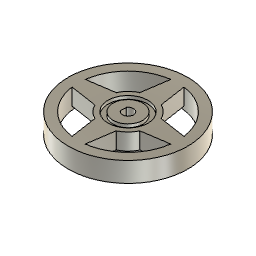
proto_wheel (Autodesk Fusion 360 design; units mm, degrees)
Autodesk Fusion 360 part; units mm, degrees
sketch "스케치1" plane through (0, 0, 0) normal (0, 0, 1) x (1, 0, 0)
  circle A0 centre (0, 0) radius 36
  dimension "d1" = 72
  constraint coincident A0.centre origin
  measures "d1" diameter of A0
extrude "돌출1" add sketch "스케치1" along normal blind 12 makes body 1
sketch "스케치2" plane through (0, 0, 12) normal (0, 0, 1) x (-1, 0, 0)
  circle A0 centre (0, 0) radius 36
  circle A1 centre (0, 0) radius 9
  circle A2 centre (0, 0) radius 12
  dimension "d4" = 18
  dimension "d5" = 24
  constraint concentric A0 A1
  constraint concentric A1 A2
  measures "d4" diameter of A1
  measures "d5" diameter of A2
extrude "돌출2" cut sketch "스케치2" against normal blind 2 contours A2 bodies 1
sketch "스케치3" plane through (0, 0, 12) normal (0, 0, 1) x (-1, 0, 0)
  circle A0 centre (0, 0) radius 9
  circle A1 centre (0, 0) radius 30
  line L0 (32, 0) -> (32, 4)
  line L1 (32, 0) -> (32, -4)
  line L2 (-4, -32) -> (0, -32)
  line L3 (4, -32) -> (0, -32)
  line L4 (-7, 9.744) -> (-4, 29.7321)
  circle A2 centre (0, 0) radius 12
  line L5 (-4, -29.7321) -> (-7, -9.7468)
  line L6 (4, -29.7321) -> (7, -9.7468)
  line L7 (29.7321, -4) -> (9.7468, -7)
  line L8 (29.7321, 4) -> (9.7468, 7)
  line L9 (-9.7468, -7) -> (-29.7321, -4)
  line L10 (4, 32) -> (0, 32)
  line L11 (7, 9.7468) -> (4, 29.7321)
  line L12 (0, 4) -> (0, 0)
  line L13 (0, 7) -> (0, 0)
  line L14 (-9.7468, 7) -> (-29.7321, 4)
  circle A3 centre (0, 0) radius 15
  dimension "d43" = 4
  dimension "d45" = 7
  dimension "d46" = 30
  constraint concentric A0 A1
  constraint vertical L0
  constraint vertical L1
  constraint horizontal L2
  constraint horizontal L3
  constraint coincident A1 L4.end
  constraint coincident A1 L5.start
  constraint coincident A2 L5.end
  constraint coincident A1 L6.start
  constraint coincident A2 L6.end
  constraint coincident A1 L7.start
  constraint coincident A2 L7.end
  constraint coincident A1 L8.start
  constraint coincident A2 L8.end
  constraint coincident A2 L9.start
  constraint coincident A1 L9.end
  constraint horizontal L10
  constraint coincident A2 L11.start
  constraint coincident A1 L11.end
  constraint vertical L12
  constraint coincident A0.centre A1.centre
  constraint vertical L13
  constraint coincident A2 L14.start
  constraint coincident A1 L14.end
  constraint concentric A2 A3
  measures "d43" distance of A0.centre L12.start
  measures "d45" distance of A0.centre L13.start
  measures "d46" diameter of A3
extrude "돌출3" cut sketch "스케치3" against normal blind 12 contours A1 L8 L11 A3 | A1 L6 L7 A3 | A1 L4 L14 A3 | A1 L5 L9 A3 bodies 1
sketch "스케치4" plane through (0, 0, 12) normal (0, 0, 1) x (-1, 0, 0)
  circle A0 centre (0, 0) radius 9
  circle A1 centre (0, 0) radius 3.5
  dimension "d49" = 7
  constraint coincident A0.centre A1.centre
  measures "d49" diameter of A1
extrude "돌출4" cut sketch "스케치4" against normal blind 12 contours A1 bodies 1
sketch "스케치5" plane through (0, 0, 12) normal (0, 0, 1) x (-1, 0, 0)
  circle A0 centre (0, 0) radius 3.5
  circle A1 centre (0, 0) radius 9
  circle A2 centre (0, 0) radius 30
  circle A3 centre (0, 0) radius 3.5
  dimension "d52" = 60
  constraint coincident A0.centre A1.centre
  measures "d52" diameter of A2
sketch "스케치6" plane through (0, 0, 0) normal (0, 0, -1) x (1, 0, 0)
  circle A0 centre (0, 0) radius 3.5
  line L0 (-4, 29.7321) -> (-6.4287, 13.5525)
  arc A1 (-6.4287, 13.5525) -> (-13.5525, 6.4287) centre (0, 0) ccw
  line L1 (-13.5525, 6.4287) -> (-29.7321, 4)
  arc A2 (-4, 29.7321) -> (-29.7321, 4) centre (0, 0) ccw
  arc A3 (29.7321, 4) -> (4, 29.7321) centre (0, 0) ccw
  line L2 (29.7321, 4) -> (13.5525, 6.4287)
  arc A4 (13.5525, 6.4287) -> (6.4284, 13.5527) centre (0, 0) ccw
  line L3 (6.4284, 13.5527) -> (4, 29.7321)
  arc A5 (-13.5525, -6.4287) -> (-6.4287, -13.5525) centre (0, 0) ccw
  line L4 (-6.4287, -13.5525) -> (-4, -29.7321)
  arc A6 (-29.7321, -4) -> (-4, -29.7321) centre (0, 0) ccw
  line L5 (-29.7321, -4) -> (-13.5525, -6.4287)
  arc A7 (4, -29.7321) -> (29.7321, -4) centre (0, 0) ccw
  line L6 (4, -29.7321) -> (6.4287, -13.5525)
  arc A8 (6.4287, -13.5525) -> (13.5525, -6.4287) centre (0, 0) ccw
  line L7 (13.5525, -6.4287) -> (29.7321, -4)
  circle A9 centre (0, 0) radius 36
  circle A10 centre (0, 0) radius 30
  dimension "d53" = 60
  constraint coincident A0.centre A1.centre
  measures "d53" diameter of A10
extrude "돌출5" cut sketch "스케치6" against normal blind 4 contours L0 A1 L1 L2 A4 L3 A5 L4 L5 L6 A8 L7 A10 bodies 1
sketch "스케치7" plane through (0, 0, 4) normal (0, 0, -1) x (1, 0, 0)
  circle A0 centre (0, 0) radius 3.5
  arc A1 (29.7321, -4) -> (29.7321, 4) centre (0, 0) ccw
  line L0 (29.7321, 4) -> (13.5525, 6.4287)
  arc A2 (13.5525, 6.4287) -> (6.4284, 13.5527) centre (0, 0) ccw
  line L1 (6.4284, 13.5527) -> (4, 29.7321)
  arc A3 (4, 29.7321) -> (-4, 29.7321) centre (0, 0) ccw
  line L2 (-4, 29.7321) -> (-6.4287, 13.5525)
  arc A4 (-6.4287, 13.5525) -> (-13.5525, 6.4287) centre (0, 0) ccw
  line L3 (-13.5525, 6.4287) -> (-29.7321, 4)
  arc A5 (-29.7321, 4) -> (-29.7321, -4) centre (0, 0) ccw
  line L4 (-29.7321, -4) -> (-13.5525, -6.4287)
  arc A6 (-13.5525, -6.4287) -> (-6.4287, -13.5525) centre (0, 0) ccw
  line L5 (-6.4287, -13.5525) -> (-4, -29.7321)
  arc A7 (-4, -29.7321) -> (4, -29.7321) centre (0, 0) ccw
  line L6 (4, -29.7321) -> (6.4287, -13.5525)
  arc A8 (6.4287, -13.5525) -> (13.5525, -6.4287) centre (0, 0) ccw
  line L7 (13.5525, -6.4287) -> (29.7321, -4)
  circle A9 centre (0, 0) radius 9
  dimension "d56" = 18
  constraint concentric A0 A9
  measures "d56" diameter of A9
extrude "돌출6" add sketch "스케치7" along normal blind 4 contours A9 bodies 1
extrude "돌출7" add 1 faces at (7.1201, 0.621, 0) along direction (0, 0, -1) blind 5 on bodies 1 bodies 1
extrude "돌출8" add sketch "스케치5" against normal blind 12 contours A0 A3 bodies 1
extrude "돌출9" add 1 faces at (-0.5349, -0.3647, 0) along direction (0, 0, -1) blind 5 on bodies 1 bodies 1
extrude "돌출10" add 1 faces at (0.4456, 19.0251, 4) along direction (0, 0, -1) blind 2 on bodies 1 bodies 1
sketch "스케치8" plane through (0, 0, -5) normal (0, 0, -1) x (1, 0, 0)
  circle A0 centre (0, 0) radius 9
  circle A1 centre (0, 0) radius 3
  dimension "d67" = 6
  constraint coincident A0.centre A1.centre
  measures "d67" diameter of A1
extrude "돌출11" cut sketch "스케치8" against normal blind 12 contours A1 bodies 1
extrude "돌출12" cut 1 faces at (-1.1591, -0.5829, 7) along direction (0, 0, 1) blind 3 on bodies 1 bodies 1
extrude "돌출13" cut 1 faces at (-1.1591, -0.5829, 10) along direction (0, 0, 1) blind 3 on bodies 1 bodies 1
sketch "스케치9" plane through (0, 0, 0) normal (0, 0, 1) x (1, 0, 0)
  line L0 (-3, 0) -> (2.5, 0)
  line L1 (2.5, 0) -> (2.5, -4)
  line L2 (2.5, -4) -> (2.5, 0)
  circle A0 centre (0, 0) radius 3
  line L3 (2.5, -1.6583) -> (3.6748, -1.6583)
  line L4 (3.6748, -1.6583) -> (3.6748, 1.7849)
  line L5 (3.6748, 1.7849) -> (2.5, 1.7849)
  line L6 (2.5, 1.7849) -> (2.5, -1.6583)
  dimension "d74" = 5.5
  dimension "d75" = 6
  constraint horizontal L0
  constraint perpendicular L0 L1
  constraint coincident A0.centre origin
  constraint horizontal L3
  constraint vertical L4
  constraint horizontal L5
  constraint vertical L6
  constraint coincident L1 L3.start
  constraint coincident A0 L3.start
  measures "d74" distance of L0.start L0.end
  measures "d75" diameter of A0
extrude "돌출14" add sketch "스케치9" along normal blind 5 contours L1 L2 A0 L6 bodies 1
extrude "돌출15" add 1 faces at (2.8226, -0.1459, 5) along direction (0, 0, 1) blind 7 on bodies 1 bodies 1
extrude "돌출16" add 1 faces at (2.8226, -0.1459, 0) along direction (0, 0, -1) blind 5 on bodies 1 bodies 1
sketch "스케치10" plane through (0, 0, -5) normal (0, 0, -1) x (1, 0, 0)
  arc A0 (2.5, 1.6583) -> (2.5, -1.6583) centre (0, 0) ccw
  line L0 (2.5, 1.6583) -> (2.5, -1.6583)
  circle A1 centre (0, 0) radius 9
  line L1 (2.5, 0) -> (3.5, 0)
  line L2 (3.5, 0) -> (6.5, 0)
  line L3 (6.5, 0) -> (6.5, 3.5)
  line L4 (6.5, 3.5) -> (3.5, 3.5)
  line L5 (3.5, 3.5) -> (3.5, 0)
  line L6 (3.5, 0) -> (6.5, 0)
  line L7 (6.5, 0) -> (6.5, -3.5)
  line L8 (6.5, -3.5) -> (3.5, -3.5)
  line L9 (3.5, -3.5) -> (3.5, 0)
  dimension "d82" = 1
  dimension "d83" = 3
  dimension "d84" = 3.5
  dimension "d85" = 3.5
  constraint midpoint L0 L1.start
  constraint perpendicular L0 L1
  constraint horizontal L2
  constraint vertical L3
  constraint horizontal L4
  constraint vertical L5
  constraint horizontal L6
  constraint vertical L7
  constraint horizontal L8
  constraint vertical L9
  measures "d82" distance of L1.start L1.end
  measures "d83" distance of L1.end L2.end
  measures "d84" distance of L1.end L4.end
  measures "d85" distance of L1.end L8.end
extrude "돌출17" cut sketch "스케치10" against normal blind 7 contours L2 L3 L4 L5 L6 | L2 L6 L7 L8 L9 bodies 1
sketch "스케치11" plane through (6.5, 0, 0) normal (-1, 0, 0) x (0, -1, 0)
  line L0 (-3.5, -5) -> (3.5, -5)
  line L1 (3.5, -5) -> (3.5, 2)
  line L2 (3.5, 2) -> (-3.5, 2)
  line L3 (-3.5, 2) -> (-3.5, -5)
  line L4 (3.5, 2) -> (0, 2)
  line L5 (3.5, -1.5) -> (3.5, 2)
  circle A0 centre (0, -1.5) radius 2.5
  dimension "d88" = 3.5
  dimension "d89" = 3.5
  dimension "d90" = 5
  constraint horizontal L4
  constraint vertical L5
  constraint coincident L1.end L2.start
  measures "d88" distance of L1.end L4.end
  measures "d89" distance of L1.end L5.start
  measures "d90" diameter of A0
extrude "돌출18" cut sketch "스케치11" against normal blind 3 contours A0 bodies 1
sketch "스케치13" plane through (3.5, 0, 0) normal (1, 0, 0) x (0, 1, 0)
  line L0 (-3.5, -5) -> (3.5, -5)
  line L1 (3.5, -5) -> (3.5, 2)
  line L2 (3.5, 2) -> (-3.5, 2)
  line L3 (-3.5, 2) -> (-3.5, -5)
  line L4 (3.5, 2) -> (0, 2)
  line L5 (0, 2) -> (0, -1.5)
  line L6 (0, -1.5) -> (3.5, -1.5)
  line L7 (3.5, -1.5) -> (3.5, 2)
  circle A0 centre (0, -1.5) radius 2.5
  dimension "d93" = 3.5
  dimension "d94" = 3.5
  dimension "d95" = 5
  constraint horizontal L4
  constraint vertical L5
  constraint horizontal L6
  constraint vertical L7
  constraint coincident L1.end L2.start
  constraint coincident L5.end L6.start
  measures "d93" distance of L1.end L4.end
  measures "d94" distance of L1.end L6.end
  measures "d95" diameter of A0
extrude "돌출19" cut sketch "스케치13" against normal blind 1 contours L5 L6 A0 | L5 L6 A0 bodies 1
extrude "돌출20" cut 1 faces at (2.5, 1.7404, -2.1634) along direction (-1, 0, 0) blind 0.4 on bodies 1 bodies 1
extrude "돌출21" cut 1 faces at (2.5, -1.7404, -2.1634) along direction (-1, 0, 0) blind 1.5 on bodies 1 bodies 1
extrude "돌출22" add 1 faces at (2.1, 2.1939, -1.1708) along direction (-1, 0, 0) blind 1.5 on bodies 1 bodies 1
extrude "돌출23" cut 1 faces at (0.6, 2.1939, -1.1708) along direction (1, 0, 0) blind 1.5 on bodies 1 bodies 1
sketch "스케치14" plane through (0, 0, -5) normal (0, 0, -1) x (1, 0, 0)
  line L0 (3.5, 3.5) -> (6.5, 3.5)
  line L1 (6.5, 3.5) -> (6.5, -3.5)
  line L2 (6.5, -3.5) -> (3.5, -3.5)
  line L3 (3.5, -3.5) -> (3.5, 3.5)
  arc A0 (2.5, 1.6583) -> (2.5, -1.6583) centre (0, 0) ccw
  line L4 (2.5, 1.6583) -> (2.5, -1.6583)
  circle A1 centre (0, 0) radius 9
  line L5 (-5, 0) -> (-5.5, 0)
  line L6 (-5.5, 0) -> (-5.5, 0.5)
  line L7 (-5.5, 0.5) -> (-5, 0.5)
  line L8 (-5, 0.5) -> (-5, 0)
  line L9 (-5, 0) -> (-5.5, 0)
  line L10 (-5.5, 0) -> (-5.5, -0.5)
  line L11 (-5.5, -0.5) -> (-5, -0.5)
  line L12 (-5, -0.5) -> (-5, 0)
  dimension "d106" = 0.5
  dimension "d107" = 0.5
  dimension "d108" = 0.5
  constraint horizontal L5
  constraint vertical L6
  constraint horizontal L7
  constraint vertical L8
  constraint horizontal L9
  constraint vertical L10
  constraint horizontal L11
  constraint vertical L12
  measures "d106" distance of L5.start L5.end
  measures "d107" distance of L5.start L7.end
  measures "d108" distance of L5.start L11.end
extrude "돌출24" cut sketch "스케치14" against normal blind 0.5 contours L5 L9 L10 L11 L12 | L5 L6 L7 L8 L9 bodies 1
sketch "스케치15" plane through (2.5, 0, 0) normal (-1, 0, 0) x (0, -1, 0)
  arc A0 (-1.6583, -3.3708) -> (1.6583, -3.3708) centre (0, -1.5) ccw
  line L0 (-1.6583, -3.3708) -> (-1.6583, -5)
  line L1 (-1.6583, -5) -> (1.6583, -5)
  line L2 (1.6583, -5) -> (1.6583, -3.3708)
  line L3 (0, -4) -> (0, 1)
  circle A1 centre (0, -1.5) radius 2.5
  dimension "d111" = 5
  dimension "d112" = 5
  constraint midpoint A0 L3.start
  constraint vertical L3
  constraint concentric A0 A1
  measures "d111" distance of L3.start L3.end
  measures "d112" diameter of A1
extrude "돌출25" add sketch "스케치15" against normal blind 1 contours A0 L3 A1 | A0 L3 A1 bodies 1
sketch "스케치16" plane through (6.5, 0, 0) normal (-1, 0, 0) x (0, -1, 0)
  circle A0 centre (0, -1.5) radius 2.5
  line L0 (-3.5, -5) -> (3.5, -5)
  line L1 (3.5, -5) -> (3.5, 2)
  line L2 (3.5, 2) -> (-3.5, 2)
  line L3 (-3.5, 2) -> (-3.5, -5)
  line L4 (0, -4) -> (0, 1)
  circle A1 centre (0, -1.5) radius 2.5
  dimension "d115" = 5
  constraint vertical L4
  constraint coincident A0 L4.start
  constraint concentric A0 A1
  measures "d115" distance of L4.start L4.end
extrude "돌출26" add sketch "스케치16" against normal blind 2 contours A0 L4 A1 | A0 L4 A1 bodies 1
sketch "스케치17" plane through (8.5, 0, 0) normal (1, 0, 0) x (0, 1, 0)
  circle A0 centre (0, -1.5) radius 2.5
  circle A1 centre (0, -1.5) radius 2
  dimension "d118" = 4
  constraint concentric A0 A1
  measures "d118" diameter of A1
extrude "돌출27" cut sketch "스케치17" against normal blind 4 contours A1 bodies 1
sketch "스케치18" plane through (3.5, 0, 0) normal (1, 0, 0) x (0, 1, 0)
  line L0 (-3.5, -5) -> (3.5, -5)
  line L1 (3.5, -5) -> (3.5, 2)
  line L2 (3.5, 2) -> (-3.5, 2)
  line L3 (-3.5, 2) -> (-3.5, -5)
  line L4 (3.5, 2) -> (0, 2)
  line L5 (0, 2) -> (0, -1.5)
  line L6 (0, -1.5) -> (3.5, -1.5)
  line L7 (3.5, -1.5) -> (3.5, 2)
  circle A0 centre (0, -1.5) radius 2
  dimension "d121" = 3.5
  dimension "d122" = 3.5
  dimension "d123" = 4
  constraint horizontal L4
  constraint vertical L5
  constraint horizontal L6
  constraint vertical L7
  constraint coincident L1.end L2.start
  constraint coincident L5.end L6.start
  measures "d121" distance of L1.end L4.end
  measures "d122" distance of L1.end L6.end
  measures "d123" diameter of A0
extrude "돌출28" cut sketch "스케치18" against normal blind 1.5 contours L5 L6 A0 | L5 L6 A0 bodies 1
sketch "스케치19" plane through (0, 0, -5) normal (0, 0, -1) x (1, 0, 0)
  line L0 (-5, -0.5) -> (-5.5, -0.5)
  line L1 (-5.5, -0.5) -> (-5.5, 0.5)
  line L2 (-5.5, 0.5) -> (-5, 0.5)
  line L3 (-5, 0.5) -> (-5, -0.5)
  line L4 (3.5, 3.5) -> (6.5, 3.5)
  line L5 (6.5, 3.5) -> (6.5, -3.5)
  line L6 (6.5, -3.5) -> (3.5, -3.5)
  line L7 (3.5, -3.5) -> (3.5, 3.5)
  arc A0 (2.5, 1.6583) -> (2.5, -1.6583) centre (0, 0) ccw
  line L8 (2.5, 1.6583) -> (2.5, -1.6583)
  circle A1 centre (0, 0) radius 9
  circle A2 centre (0, 0) radius 3
  dimension "d126" = 6
  constraint coincident A0.centre A1.centre
  measures "d126" diameter of A2
extrude "돌출29" add sketch "스케치19" against normal blind 17 contours A0 L8 A2 bodies 1
extrude "돌출30" add 1 faces at (-5.3333, 0.1667, -4.5) along direction (0, 0, -1) blind 0.5 on bodies 1 bodies 1
sketch "스케치20" plane through (0, 0, -5) normal (0, 0, -1) x (1, 0, 0)
  line L0 (3.5, 3.5) -> (6.5, 3.5)
  line L1 (6.5, 3.5) -> (6.5, -3.5)
  line L2 (6.5, -3.5) -> (3.5, -3.5)
  line L3 (3.5, -3.5) -> (3.5, 3.5)
  circle A0 centre (0, 0) radius 9
  circle A1 centre (0, 0) radius 9
  constraint coincident A0.centre A1.centre
extrude "돌출31" cut sketch "스케치20" against normal blind 7 contours L0 L1 L2 L3 | A0 A1 bodies 1
sketch "스케치21" plane through (0, 0, 2) normal (0, 0, -1) x (1, 0, 0)
  arc A0 (29.7321, -4) -> (29.7321, 4) centre (0, 0) ccw
  line L0 (29.7321, 4) -> (13.5525, 6.4287)
  arc A1 (13.5525, 6.4287) -> (6.4284, 13.5527) centre (0, 0) ccw
  line L1 (6.4284, 13.5527) -> (4, 29.7321)
  arc A2 (4, 29.7321) -> (-4, 29.7321) centre (0, 0) ccw
  line L2 (-4, 29.7321) -> (-6.4287, 13.5525)
  arc A3 (-6.4287, 13.5525) -> (-13.5525, 6.4287) centre (0, 0) ccw
  line L3 (-13.5525, 6.4287) -> (-29.7321, 4)
  arc A4 (-29.7321, 4) -> (-29.7321, -4) centre (0, 0) ccw
  line L4 (-29.7321, -4) -> (-13.5525, -6.4287)
  arc A5 (-13.5525, -6.4287) -> (-6.4287, -13.5525) centre (0, 0) ccw
  line L5 (-6.4287, -13.5525) -> (-4, -29.7321)
  arc A6 (-4, -29.7321) -> (4, -29.7321) centre (0, 0) ccw
  line L6 (4, -29.7321) -> (6.4287, -13.5525)
  arc A7 (6.4287, -13.5525) -> (13.5525, -6.4287) centre (0, 0) ccw
  line L7 (13.5525, -6.4287) -> (29.7321, -4)
  circle A8 centre (0, 0) radius 10
  dimension "d133" = 20
  constraint coincident A0.centre A1.centre
  measures "d133" diameter of A8
extrude "돌출32" add sketch "스케치21" along normal blind 7 contours A8 bodies 1
sketch "스케치22" plane through (0, 0, -5) normal (0, 0, -1) x (1, 0, 0)
  circle A0 centre (0, 0) radius 10
  circle A1 centre (0, 0) radius 3.15
  line L0 (-3.15, -0.0084) -> (2.65, -0.0084)
  line L1 (2.65, -0.0084) -> (3.4893, -0.0084)
  line L2 (3.4893, -0.0084) -> (3.4893, -2.2916)
  line L3 (3.4893, -2.2916) -> (2.65, -2.2916)
  line L4 (2.65, -2.2916) -> (2.65, -0.0084)
  line L5 (2.65, -0.0084) -> (3.8352, -0.0084)
  line L6 (3.8352, -0.0084) -> (3.8352, 2.5515)
  line L7 (3.8352, 2.5515) -> (2.65, 2.5515)
  line L8 (2.65, 2.5515) -> (2.65, -0.0084)
  dimension "d136" = 6.3
  dimension "d137" = 5.8
  constraint coincident A0.centre A1.centre
  constraint coincident A1 L0.start
  constraint horizontal L0
  constraint horizontal L1
  constraint vertical L2
  constraint horizontal L3
  constraint vertical L4
  constraint horizontal L5
  constraint vertical L6
  constraint horizontal L7
  constraint vertical L8
  measures "d136" diameter of A1
  measures "d137" distance of L0.start L0.end
extrude "돌출33" cut sketch "스케치22" against normal blind 16 contours A1 L0 L8 | A1 L0 L4 bodies 1
extrude "돌출34" cut 1 faces at (-1.2063, -0.1412, 11) along direction (0, 0, 1) blind 1 on bodies 1 bodies 1
sketch "스케치23" plane through (0, 0, -5) normal (0, 0, -1) x (1, 0, 0)
  line L0 (2.65, 1.7029) -> (2.65, -1.7029)
  arc A0 (2.65, 1.7029) -> (2.65, -1.7029) centre (0, 0) ccw
  circle A1 centre (0, 0) radius 10
  line L1 (2.65, 0) -> (3.65, 0)
  line L2 (3.65, 0) -> (7.65, 0)
  line L3 (7.65, 0) -> (7.65, -3.5)
  line L4 (7.65, -3.5) -> (3.65, -3.5)
  line L5 (3.65, -3.5) -> (3.65, 0)
  line L6 (3.65, 0) -> (7.65, 0)
  line L7 (7.65, 0) -> (7.65, 3.5)
  line L8 (7.65, 3.5) -> (3.65, 3.5)
  line L9 (3.65, 3.5) -> (3.65, 0)
  dimension "d142" = 1
  dimension "d143" = 4
  dimension "d144" = 3.5
  dimension "d145" = 3.5
  constraint midpoint L0 L1.start
  constraint perpendicular L0 L1
  constraint horizontal L2
  constraint vertical L3
  constraint horizontal L4
  constraint vertical L5
  constraint horizontal L6
  constraint vertical L7
  constraint horizontal L8
  constraint vertical L9
  measures "d142" distance of L1.start L1.end
  measures "d143" distance of L1.end L2.end
  measures "d144" distance of L1.end L4.end
  measures "d145" distance of L1.end L8.end
extrude "돌출35" cut sketch "스케치23" against normal blind 7 contours L2 L6 L7 L8 L9 | L2 L3 L4 L5 L6 bodies 1
sketch "스케치24" plane through (0, 0, -5) normal (0, 0, -1) x (1, 0, 0)
  line L0 (3.65, 3.5) -> (7.65, 3.5)
  line L1 (7.65, 3.5) -> (7.65, -3.5)
  line L2 (7.65, -3.5) -> (3.65, -3.5)
  line L3 (3.65, -3.5) -> (3.65, 3.5)
  line L4 (2.65, 1.7029) -> (2.65, -1.7029)
  arc A0 (2.65, 1.7029) -> (2.65, -1.7029) centre (0, 0) ccw
  circle A1 centre (0, 0) radius 10
  line L5 (0, -6) -> (-0.5, -6)
  line L6 (-0.5, -6) -> (-0.5, -6.5)
  line L7 (-0.5, -6.5) -> (0, -6.5)
  line L8 (0, -6.5) -> (0, -6)
  line L9 (0, -6) -> (0.5, -6)
  line L10 (0.5, -6) -> (0.5, -6.5)
  line L11 (0.5, -6.5) -> (0, -6.5)
  line L12 (0, -6.5) -> (0, -6)
  dimension "d148" = 0.5
  dimension "d149" = 0.5
  dimension "d150" = 0.5
  constraint horizontal L5
  constraint vertical L6
  constraint horizontal L7
  constraint vertical L8
  constraint horizontal L9
  constraint vertical L10
  constraint horizontal L11
  constraint vertical L12
  measures "d148" distance of L5.start L5.end
  measures "d149" distance of L5.start L7.end
  measures "d150" distance of L5.start L7.end
extrude "돌출36" cut sketch "스케치24" against normal blind 0.5 contours L5 L6 L7 L8 L12 | L8 L9 L10 L11 L12 bodies 1
sketch "스케치25" plane through (3.65, 0, 0) normal (1, 0, 0) x (0, 1, 0)
  line L0 (-3.5, -5) -> (3.5, -5)
  line L1 (3.5, -5) -> (3.5, 2)
  line L2 (3.5, 2) -> (-3.5, 2)
  line L3 (-3.5, 2) -> (-3.5, -5)
  line L4 (3.5, 2) -> (0, 2)
  line L5 (0, 2) -> (0, -1.5)
  line L6 (0, -1.5) -> (3.5, -1.5)
  line L7 (3.5, -1.5) -> (3.5, 2)
  circle A0 centre (0, -1.5) radius 2
  dimension "d153" = 3.5
  dimension "d154" = 3.5
  dimension "d155" = 4
  constraint horizontal L4
  constraint vertical L5
  constraint horizontal L6
  constraint vertical L7
  constraint coincident L1.end L2.start
  constraint coincident L5.end L6.start
  measures "d153" distance of L1.end L4.end
  measures "d154" distance of L1.end L6.end
  measures "d155" diameter of A0
extrude "돌출37" cut sketch "스케치25" against normal blind 3.5 contours L5 L6 A0 | L5 L6 A0 bodies 1
sketch "스케치26" plane through (7.65, 0, 0) normal (-1, 0, 0) x (0, -1, 0)
  line L0 (-3.5, -5) -> (3.5, -5)
  line L1 (3.5, -5) -> (3.5, 2)
  line L2 (3.5, 2) -> (-3.5, 2)
  line L3 (-3.5, 2) -> (-3.5, -5)
  line L4 (3.5, 2) -> (0, 2)
  line L5 (0, 2) -> (0, -1.5)
  line L6 (0, -1.5) -> (3.5, -1.5)
  line L7 (3.5, -1.5) -> (3.5, 2)
  circle A0 centre (0, -1.5) radius 2
  dimension "d158" = 3.5
  dimension "d159" = 3.5
  dimension "d160" = 4
  constraint horizontal L4
  constraint vertical L5
  constraint horizontal L6
  constraint vertical L7
  constraint coincident L1.end L2.start
  constraint coincident L5.end L6.start
  measures "d158" distance of L1.end L4.end
  measures "d159" distance of L1.end L6.end
  measures "d160" diameter of A0
extrude "돌출38" cut sketch "스케치26" against normal blind 3.5 contours L5 L6 A0 | L5 L6 A0 bodies 1
extrude "돌출39" cut 1 faces at (3.05, 6.2201, -5) along direction (0, 0, 1) blind 7 on bodies 1 bodies 1
extrude "돌출40" cut 1 faces at (-0.1667, 6.3333, -4.5) along direction (0, 0, 1) blind 6.5 on bodies 1 bodies 1
sketch "스케치27" plane through (0, 0, 2) normal (0, 0, -1) x (1, 0, 0)
  arc A0 (29.7321, -4) -> (29.7321, 4) centre (0, 0) ccw
  line L0 (29.7321, 4) -> (13.5525, 6.4287)
  arc A1 (13.5525, 6.4287) -> (6.4284, 13.5527) centre (0, 0) ccw
  line L1 (6.4284, 13.5527) -> (4, 29.7321)
  arc A2 (4, 29.7321) -> (-4, 29.7321) centre (0, 0) ccw
  line L2 (-4, 29.7321) -> (-6.4287, 13.5525)
  arc A3 (-6.4287, 13.5525) -> (-13.5525, 6.4287) centre (0, 0) ccw
  line L3 (-13.5525, 6.4287) -> (-29.7321, 4)
  arc A4 (-29.7321, 4) -> (-29.7321, -4) centre (0, 0) ccw
  line L4 (-29.7321, -4) -> (-13.5525, -6.4287)
  arc A5 (-13.5525, -6.4287) -> (-6.4287, -13.5525) centre (0, 0) ccw
  line L5 (-6.4287, -13.5525) -> (-4, -29.7321)
  arc A6 (-4, -29.7321) -> (4, -29.7321) centre (0, 0) ccw
  line L6 (4, -29.7321) -> (6.4287, -13.5525)
  arc A7 (6.4287, -13.5525) -> (13.5525, -6.4287) centre (0, 0) ccw
  line L7 (13.5525, -6.4287) -> (29.7321, -4)
  line L8 (2.65, 1.7029) -> (2.65, -1.7029)
  arc A8 (2.65, 1.7029) -> (2.65, -1.7029) centre (0, 0) ccw
  circle A9 centre (0, 0) radius 11
  dimension "d167" = 22
  constraint coincident A0.centre A1.centre
  measures "d167" diameter of A9
extrude "돌출41" add sketch "스케치27" against normal blind 10 contours L8 A8 bodies 1
sketch "스케치28" plane through (0, 0, 2) normal (0, 0, -1) x (1, 0, 0)
  arc A0 (29.7321, -4) -> (29.7321, 4) centre (0, 0) ccw
  line L0 (29.7321, 4) -> (13.5525, 6.4287)
  arc A1 (13.5525, 6.4287) -> (6.4284, 13.5527) centre (0, 0) ccw
  line L1 (6.4284, 13.5527) -> (4, 29.7321)
  arc A2 (4, 29.7321) -> (-4, 29.7321) centre (0, 0) ccw
  line L2 (-4, 29.7321) -> (-6.4287, 13.5525)
  arc A3 (-6.4287, 13.5525) -> (-13.5525, 6.4287) centre (0, 0) ccw
  line L3 (-13.5525, 6.4287) -> (-29.7321, 4)
  arc A4 (-29.7321, 4) -> (-29.7321, -4) centre (0, 0) ccw
  line L4 (-29.7321, -4) -> (-13.5525, -6.4287)
  arc A5 (-13.5525, -6.4287) -> (-6.4287, -13.5525) centre (0, 0) ccw
  line L5 (-6.4287, -13.5525) -> (-4, -29.7321)
  arc A6 (-4, -29.7321) -> (4, -29.7321) centre (0, 0) ccw
  line L6 (4, -29.7321) -> (6.4287, -13.5525)
  arc A7 (6.4287, -13.5525) -> (13.5525, -6.4287) centre (0, 0) ccw
  line L7 (13.5525, -6.4287) -> (29.7321, -4)
  circle A8 centre (0, 0) radius 11
  dimension "d170" = 22
  constraint concentric A0 A8
  measures "d170" diameter of A8
extrude "돌출42" add sketch "스케치28" along normal blind 7 contours A8 bodies 1
sketch "스케치29" plane through (0, 0, -5) normal (0, 0, -1) x (1, 0, 0)
  circle A0 centre (0, 0) radius 11
  circle A1 centre (0, 0) radius 3.3
  line L0 (3.3, 0.0071) -> (-2.8, 0.0071)
  line L1 (-2.8, 0.0071) -> (-3.7029, 0.0071)
  line L2 (-3.7029, 0.0071) -> (-3.7029, -2.254)
  line L3 (-3.7029, -2.254) -> (-2.8, -2.254)
  line L4 (-2.8, -2.254) -> (-2.8, 0.0071)
  line L5 (-2.8, 0.0071) -> (-4, 0.0071)
  line L6 (-4, 0.0071) -> (-4, 2.5)
  line L7 (-4, 2.5) -> (-2.8, 2.5)
  line L8 (-2.8, 2.5) -> (-2.8, 0.0071)
  dimension "d173" = 6.6
  dimension "d174" = 6.1
  constraint coincident A0.centre A1.centre
  constraint coincident A1 L0.start
  constraint horizontal L0
  constraint horizontal L1
  constraint vertical L2
  constraint horizontal L3
  constraint vertical L4
  constraint horizontal L5
  constraint vertical L6
  constraint horizontal L7
  constraint vertical L8
  measures "d173" diameter of A1
  measures "d174" distance of L0.start L0.end
extrude "돌출43" cut sketch "스케치29" against normal blind 17 contours A1 L0 L4 | A1 L0 L8 bodies 1
sketch "스케치30" plane through (0, 0, -5) normal (0, 0, -1) x (1, 0, 0)
  line L0 (-2.8, -1.7464) -> (-2.8, 1.7464)
  arc A0 (-2.8, -1.7464) -> (-2.8, 1.7464) centre (0, 0) ccw
  circle A1 centre (0, 0) radius 11
  line L1 (-0.0206, -5.7223) -> (-0.5206, -5.7223)
  line L2 (-0.5206, -5.7223) -> (-0.5206, -6.2223)
  line L3 (-0.5206, -6.2223) -> (-0.0206, -6.2223)
  line L4 (-0.0206, -6.2223) -> (-0.0206, -5.7223)
  line L5 (-0.0206, -5.7223) -> (0.4794, -5.7223)
  line L6 (0.4794, -5.7223) -> (0.4794, -6.2223)
  line L7 (0.4794, -6.2223) -> (-0.0206, -6.2223)
  line L8 (-0.0206, -6.2223) -> (-0.0206, -5.7223)
  dimension "d177" = 0.5
  dimension "d178" = 0.5
  dimension "d179" = 0.5
  constraint horizontal L1
  constraint vertical L2
  constraint horizontal L3
  constraint vertical L4
  constraint horizontal L5
  constraint vertical L6
  constraint horizontal L7
  constraint vertical L8
  measures "d177" distance of L1.start L1.end
  measures "d178" distance of L1.start L3.end
  measures "d179" distance of L1.start L3.end
extrude "돌출44" cut sketch "스케치30" against normal blind 0.5 contours L1 L2 L3 L4 L8 | L4 L5 L6 L7 L8 bodies 1
sketch "스케치31" plane through (0, 0, -5) normal (0, 0, -1) x (1, 0, 0)
  line L0 (-0.5206, -6.2223) -> (-0.5206, -5.7223)
  line L1 (-0.5206, -5.7223) -> (0.4794, -5.7223)
  line L2 (0.4794, -5.7223) -> (0.4794, -6.2223)
  line L3 (0.4794, -6.2223) -> (-0.5206, -6.2223)
  line L4 (-2.8, -1.7464) -> (-2.8, 1.7464)
  arc A0 (-2.8, -1.7464) -> (-2.8, 1.7464) centre (0, 0) ccw
  circle A1 centre (0, 0) radius 11
  line L5 (-2.8, 0) -> (-4.3, 0)
  line L6 (-4.3, 0) -> (-8.3, 0)
  line L7 (-8.3, 0) -> (-8.3, -3.5)
  line L8 (-8.3, -3.5) -> (-4.3, -3.5)
  line L9 (-4.3, -3.5) -> (-4.3, 0)
  line L10 (-4.3, 0) -> (-8.3, 0)
  line L11 (-8.3, 0) -> (-8.3, 3.5)
  line L12 (-8.3, 3.5) -> (-4.3, 3.5)
  line L13 (-4.3, 3.5) -> (-4.3, 0)
  dimension "d182" = 1.5
  dimension "d183" = 4
  dimension "d184" = 3.5
  dimension "d185" = 3.5
  constraint midpoint L4 L5.start
  constraint perpendicular L4 L5
  constraint horizontal L6
  constraint vertical L7
  constraint horizontal L8
  constraint vertical L9
  constraint horizontal L10
  constraint vertical L11
  constraint horizontal L12
  constraint vertical L13
  measures "d182" distance of L5.start L5.end
  measures "d183" distance of L5.end L6.end
  measures "d184" distance of L5.end L8.end
  measures "d185" distance of L5.end L12.end
extrude "돌출45" cut sketch "스케치31" against normal blind 7 contours L6 L7 L8 L9 L10 | L6 L10 L11 L12 L13 bodies 1
sketch "스케치32" plane through (-4.3, 0, 0) normal (-1, 0, 0) x (0, -1, 0)
  line L0 (-3.5, -5) -> (3.5, -5)
  line L1 (3.5, -5) -> (3.5, 2)
  line L2 (3.5, 2) -> (-3.5, 2)
  line L3 (-3.5, 2) -> (-3.5, -5)
  line L4 (3.5, 2) -> (0, 2)
  line L5 (0, 2) -> (0, -1.5)
  line L6 (0, -1.5) -> (3.5, -1.5)
  line L7 (3.5, -1.5) -> (3.5, 2)
  circle A0 centre (0, -1.5) radius 2
  line L8 (-2.3389, -7.6323) -> (1.1611, -7.6323)
  line L9 (1.1611, -7.6323) -> (1.1611, -11.1323)
  line L10 (1.1611, -11.1323) -> (-2.3389, -11.1323)
  line L11 (-2.3389, -11.1323) -> (-2.3389, -7.6323)
  dimension "d188" = 3.5
  dimension "d189" = 3.5
  dimension "d190" = 4
  dimension "d191" = 3.5
  dimension "d192" = 3.5
  constraint horizontal L4
  constraint vertical L5
  constraint horizontal L6
  constraint vertical L7
  constraint coincident L1.end L2.start
  constraint coincident L5.end L6.start
  constraint horizontal L8
  constraint vertical L9
  constraint horizontal L10
  constraint vertical L11
  measures "d188" distance of L1.end L4.end
  measures "d189" distance of L1.end L6.end
  measures "d190" diameter of A0
  measures "d191" distance of L8.start L8.end
  measures "d192" distance of L8.start L10.end
extrude "돌출46" cut sketch "스케치32" against normal blind 5 contours L5 L6 A0 | L5 L6 A0 bodies 1
sketch "스케치33" plane through (-8.3, 0, 0) normal (1, 0, 0) x (0, 1, 0)
  line L0 (-3.5, -5) -> (3.5, -5)
  line L1 (3.5, -5) -> (3.5, 2)
  line L2 (3.5, 2) -> (-3.5, 2)
  line L3 (-3.5, 2) -> (-3.5, -5)
  line L4 (3.5, 2) -> (0, 2)
  line L5 (0, 2) -> (0, -1.5)
  line L6 (0, -1.5) -> (3.5, -1.5)
  line L7 (3.5, -1.5) -> (3.5, 2)
  circle A0 centre (0, -1.5) radius 2
  dimension "d195" = 3.5
  dimension "d196" = 3.5
  dimension "d197" = 4
  constraint horizontal L4
  constraint vertical L5
  constraint horizontal L6
  constraint vertical L7
  constraint coincident L1.end L2.start
  constraint coincident L5.end L6.start
  measures "d195" distance of L1.end L4.end
  measures "d196" distance of L1.end L6.end
  measures "d197" diameter of A0
extrude "돌출47" cut sketch "스케치33" against normal blind 4.5 contours L5 L6 A0 | L5 L6 A0 bodies 1
copy_body "본체->구성요소1" bodies 1 removing the originals makes body 2 in component "Component"
component "Component" placed x (1, 0, 0) y (0, 1, 0) z (0, 0, 1) at (0, 0, 0)
